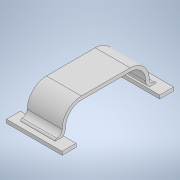
# Autodesk Inventor part: AttachmentBracket
Saved by Autodesk Inventor 2022 (Build 260153000, 153)
## iProperties
Created: 2022-02-15
Part Number: AttachmentBracket
Material: Generic
Document SubType Name: Modeling
Designer: tagaz
Density: 1 g/cm^3
Appearance: Default
Author: tagaz
Autodesk Inventor part; units mm, degrees
ref_plane "YZ Plane" through (0, 0, 0) normal (1, 0, 0) x (0, 1, 0)
ref_plane "XZ Plane" through (0, 0, 0) normal (0, 1, 0) x (-1, 0, 0)
ref_plane "XY Plane" through (0, 0, 0) normal (0, 0, 1) x (1, 0, 0)
sketch "Sketch1" plane through (0, 0, 0) normal (0, 1, 0) x (-1, 0, 0)
  line L0 (0, 0) -> (101.6, 0)
  line L1 (101.6, 0) -> (101.6, -25.4)
  line L2 (101.6, -25.4) -> (0, -25.4)
  line L3 (0, -25.4) -> (0, 0)
  line L4 (0, -177.8) -> (101.6, -177.8)
  line L5 (101.6, -177.8) -> (101.6, -203.2)
  line L6 (101.6, -203.2) -> (0, -203.2)
  line L7 (0, -203.2) -> (0, -177.8)
  point P0 (0, -190.5)
  point P1 (0, -12.7)
  dimension "d0" = 101.6
  dimension "d1" = 25.4
  dimension "d2" = 101.6
  dimension "d3" = 25.4
  dimension "d4" = 152.4
  constraints: 16 end point, 4 parallel, 2 horizontal, 2 midpoint, 2 perpendicular, 1 vertical alignment
  measures "d0" distance of L1.end L2.end
  measures "d1" distance of L0.end L1.end
  measures "d2" distance of L5.end L6.end
  measures "d3" distance of L4.end L5.end
  measures "d4" distance between parallel lines of L2 L4
extrude "Extrusion1" add sketch "Sketch1" along normal blind 6.35
ref_plane "Work Plane1" through (-50.8, 0, 0) normal (1, 0, 0) x (0, 0, -1)
sketch "Sketch2" plane through (-50.8, 0, 0) normal (1, 0, 0) x (0, 0, -1)
  line L0 (177.8, 19.05) -> (177.8, 19.05)
  line L1 (146.05, 50.8) -> (57.15, 50.8)
  line L2 (25.4, 19.05) -> (25.4, 19.05)
  arc A0 (57.15, 50.8) -> (25.4, 19.05) centre (57.15, 19.05) ccw
  arc A1 (177.8, 19.05) -> (146.05, 50.8) centre (146.05, 19.05) ccw
  line L3 (0, 6.35) -> (25.4, 6.35) projected
  arc A2 (12.7, 6.35) -> (25.4, 19.05) centre (12.7, 19.05) ccw
  line L4 (177.8, 0) -> (177.8, 6.35) projected
  line L5 (203.2, 0) -> (203.2, 6.35) projected
  arc A3 (177.8, 19.05) -> (190.5, 6.35) centre (190.5, 19.05) ccw
  point P0 (0, 0)
  point P1 (177.8, 50.8)
  point P2 (25.4, 50.8)
  dimension "d7" = 152.4
  dimension "d8" = 44.45
  dimension "d9" = 31.75
  dimension "d10" = 12.7
  dimension "d11" = 12.7
  constraints: 8 point on circle, 6 end point, 6 point on line, 6 tangent, 4 centre point, 1 equal radius, 1 parallel
  measures "d7" distance of point (25.4, 50.8) point (177.8, 50.8)
  measures "d8" distance of point (177.8, 50.8) L4.end
  measures "d9" radius of A0
  measures "d10" radius of A2
  measures "d11" radius of A3
ref_plane "Work Plane2" through (-50.8, 6.35, -12.7) normal (0, 0, 1) x (1, 0, 0)
sketch "Sketch4" plane through (-50.8, 6.35, -12.7) normal (0, 0, 1) x (1, 0, 0)
  line L0 (-34.925, -3.175) -> (28.575, -3.175)
  line L1 (28.575, -3.175) -> (28.575, 3.175)
  line L2 (28.575, 3.175) -> (-34.925, 3.175)
  line L3 (-34.925, 3.175) -> (-34.925, -3.175)
  line L4 (-50.8, 0) -> (50.8, 0) projected
  point P0 (50.8, -6.35)
  point P1 (-3.175, -3.175)
  point P2 (0, 0)
  point P3 (-3.175, 3.175)
  point P4 (-34.925, 0)
  dimension "d14" = 63.5
  dimension "d15" = 6.35
  dimension "d19" = 15.875
  constraints: 8 end point, 4 midpoint, 2 parallel, 1 horizontal, 1 horizontal alignment, 1 perpendicular
  measures "d14" distance of L2.end L1.end
  measures "d15" distance of L1.end L0.end
  measures "d19" distance from line of L4.start L3
sweep "Sweep1" add profiles "Sketch4" path "Sketch2" path curves A2 A0 L1 A1 A3
sketch "Sketch5" plane through (-85.725, 9.525, -12.7) normal (0, 0, 1) x (1, 0, 0)
  line L0 (63.5, -3.175) -> (0, -3.175) projected
  line L1 (63.5, -3.175) -> (63.5, 0) projected
  line L2 (63.5, 0) -> (0, 0) projected
  line L3 (0, 0) -> (0, -3.175) projected
  point P0 (85.725, -9.525)
revolve "Revolution1" add sketch "Sketch5" angle 90 about axis through (-22.225, 6.35, -12.7) along (1, 0, 0)
sketch "Sketch6" plane through (-22.225, 6.35, -190.5) normal (0, 0, -1) x (-1, 0, 0)
  line L0 (63.5, 0) -> (0, 0) projected
  line L1 (63.5, 0) -> (63.5, 3.175) projected
  line L2 (63.5, 3.175) -> (0, 3.175) projected
  line L3 (0, 3.175) -> (0, 0) projected
  point P0 (-22.225, -6.35)
revolve "Revolution2" add sketch "Sketch6" angle 90 about axis through (-85.725, 6.35, -190.5) along (-1, 0, 0)
body "Solid1"
